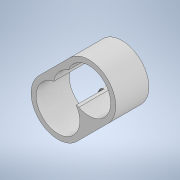
# Autodesk Inventor part: Part4
Saved by Autodesk Inventor 2020 (Build 240168000, 168)
## iProperties
Created: 2020-02-11
Part Number: Part4
Material: Generic
Document SubType Name: Modeling
Designer: atmat
Density: 1 g/cm^3
Appearance: Default
Author: atmat
Autodesk Inventor part; units mm, degrees
ref_plane "YZ Plane" through (0, 0, 0) normal (1, 0, 0) x (0, 1, 0)
ref_plane "XZ Plane" through (0, 0, 0) normal (0, 1, 0) x (-1, 0, 0)
ref_plane "XY Plane" through (0, 0, 0) normal (0, 0, 1) x (1, 0, 0)
sketch "Sketch1" plane through (0, 0, 0) normal (0, 0, 1) x (1, 0, 0)
  circle A0 centre (0, 0) radius 12.35
  circle A1 centre (7.4246, 7.4246) radius 12.2
  line L0 (-13.413, -13.413) -> (25.4094, 25.4094) construction
  line L1 (-10.6165, 0) -> (15.2552, 0) construction
  line L2 (7.4246, 7.4246) -> (15.8638, 6.41) construction
  line L3 (16.6649, 18.5138) -> (22.6753, 24.5242) construction
  circle A2 centre (15.8638, 6.41) radius 1.5
  line L4 (7.4246, 7.4246) -> (-1.0146, 8.4392) construction
  circle A3 centre (-1.0146, 8.4392) radius 1.5
  line L5 (0, 0) -> (-1.0146, 8.4392) construction
  line L6 (0, 0) -> (1.0146, -8.4392) construction
  circle A4 centre (1.0146, -8.4392) radius 1.5
  circle A5 centre (-9.8288, -9.8288) radius 12.2
  line L7 (-5.2409, -11.1828) -> (0, 0)
  point P0 (11.6813, -4.0087)
  point P1 (-0.7603, -1.6223)
  dimension "d0" = 24.7
  dimension "d1" = 24.4
  dimension "d2" = 0
  dimension "d3" = 45
  dimension "d4" = 0
  dimension "d5" = 10.5
  dimension "d20" = 8.5
  dimension "d21" = 3
  dimension "d22" = 3
  dimension "d23" = 3
  dimension "d24" = 24.4
  dimension "d25" = 24.4
  dimension "d26" = 4.5
  constraints: 18 end point, 5 centre point, 4 coincident, 4 equal length, 2 collinear, 1 horizontal, 3 other
  measures "d1" diameter of A1
  measures "d2" distance from line of point (0, 0) L0
  measures "d3" angle of L1 L0
  measures "d4" distance from line of L0 L2.start
  measures "d5" distance of point (0, 0) L2.start
  measures "d20" distance of L3.start L3.end
  measures "d21" diameter of A2
  measures "d22" diameter of A3
  measures "d23" diameter of A4
  measures "d24" diameter of A5
  measures "d25" distance of L2.start A5.centre
  measures "d26" distance from line of L7 L6.end
extrude "Extrusion1" add sketch "Sketch1" along normal blind 3 contours A0 A5 A4 L7 A1 | A0 L7 A5 A4
sketch "Sketch3" plane through (0, 0, 3) normal (0, 0, 1) x (1, 0, 0)
  circle A0 centre (0, 0) radius 12.35
  circle A1 centre (7.4246, 7.4246) radius 12.2
  line L0 (-13.413, -13.413) -> (25.4094, 25.4094) construction
  line L1 (-10.6165, 0) -> (15.2552, 0) construction
  line L2 (7.4246, 7.4246) -> (15.8638, 6.41) construction
  line L3 (16.6649, 18.5138) -> (22.6753, 24.5242) construction
  circle A2 centre (15.8638, 6.41) radius 1.5
  line L4 (7.4246, 7.4246) -> (-1.0146, 8.4392) construction
  circle A3 centre (-1.0146, 8.4392) radius 1.5
  line L5 (0, 0) -> (-1.0146, 8.4392) construction
  line L6 (0, 0) -> (1.0146, -8.4392) construction
  circle A4 centre (1.0146, -8.4392) radius 1.5
  circle A5 centre (-9.8288, -9.8288) radius 12.2
  line L7 (-5.2409, -11.1828) -> (0, 0)
  point P0 (11.6813, -4.0087)
  point P1 (-0.7603, -1.6223)
  point P2 (-0.7743, -1.6522)
  point P3 (2.1356, -7.4425)
  point P4 (2.3507, -9.1211)
  point P5 (2.146, -12.1621)
  dimension "d32" = 24.7
  dimension "d33" = 24.4
  dimension "d34" = 0
  dimension "d35" = 45
  dimension "d36" = 0
  dimension "d37" = 10.5
  dimension "d38" = 8.5
  dimension "d39" = 3
  dimension "d40" = 3
  dimension "d41" = 3
  dimension "d42" = 24.4
  dimension "d43" = 24.4
  dimension "d44" = 4.5
  constraints: 18 end point, 5 centre point, 4 coincident, 4 equal length, 2 collinear, 1 horizontal, 3 other
  measures "d33" diameter of A1
  measures "d34" distance from line of point (0, 0) L0
  measures "d35" angle of L1 L0
  measures "d36" distance from line of L0 L2.start
  measures "d37" distance of point (0, 0) L2.start
  measures "d38" distance of L3.start L3.end
  measures "d39" diameter of A2
  measures "d40" diameter of A3
  measures "d41" diameter of A4
  measures "d42" diameter of A5
  measures "d43" distance of L2.start A5.centre
  measures "d44" distance from line of L7 L6.end
extrude "Extrusion3" add sketch "Sketch3" along normal blind 15.5 contours A0 A5 A4 L7 A1 | A4 A5 picked at (2.3363, -8.2121)
sketch "Sketch4" plane through (0, 0, 3) normal (0, 0, 1) x (1, 0, 0)
  line L0 (-2.1493, -8.7099) -> (-0.8017, -5.8346)
  line L1 (-0.8017, -5.8346) -> (2.3621, -5.5639)
  line L2 (2.3621, -5.5639) -> (4.1785, -8.1686)
  line L3 (4.1785, -8.1686) -> (2.8309, -11.0439)
  line L4 (2.8309, -11.0439) -> (-0.3329, -11.3146)
  line L5 (-0.3329, -11.3146) -> (-2.1493, -8.7099)
  point P0 (0, 0)
  point P1 (1.0146, -8.4392)
  dimension "d49" = 5.5
  constraints: 12 end point, 13 other
  measures "d49" distance between parallel lines of L3 L0
extrude "Extrusion4" cut sketch "Sketch4" along normal blind 2 and the other way blind 1
sketch "Sketch5" plane through (0, 0, 18.5) normal (0, 0, 1) x (1, 0, 0)
  circle A0 centre (0, 0) radius 12.35
  circle A1 centre (7.4246, 7.4246) radius 12.2
  line L0 (-13.413, -13.413) -> (25.4094, 25.4094) construction
  line L1 (-10.6165, 0) -> (15.2552, 0) construction
  line L2 (7.4246, 7.4246) -> (15.8638, 6.41) construction
  line L3 (16.6649, 18.5138) -> (22.6753, 24.5242) construction
  circle A2 centre (15.8638, 6.41) radius 1.5
  line L4 (7.4246, 7.4246) -> (-1.0146, 8.4392) construction
  circle A3 centre (-1.0146, 8.4392) radius 1.5
  line L5 (0, 0) -> (-1.0146, 8.4392) construction
  line L6 (0, 0) -> (1.0146, -8.4392) construction
  circle A4 centre (1.0146, -8.4392) radius 1.5
  circle A5 centre (-9.8288, -9.8288) radius 12.2
  line L7 (-5.2409, -11.1828) -> (0, 0)
  line L8 (-31.042, -9.8288) -> (7.4246, 28.6378)
  line L9 (7.4246, 28.6378) -> (28.6378, 7.4246)
  line L10 (28.6378, 7.4246) -> (-9.8288, -31.042)
  line L11 (-9.8288, -31.042) -> (-31.042, -9.8288)
  circle A6 centre (-9.8288, -9.8288) radius 15
  circle A7 centre (7.4246, 7.4246) radius 15
  point P0 (11.6813, -4.0087)
  point P1 (-0.7603, -1.6223)
  point P2 (2.146, -12.1621)
  point P3 (-12.1621, 2.146)
  point P4 (-4.0087, 11.6813)
  point P5 (0.7778, -20.4354)
  point P6 (18.0312, -3.182)
  point P7 (-3.182, 18.0312)
  point P8 (-20.4354, 0.7778)
  dimension "d54" = 24.7
  dimension "d55" = 24.4
  dimension "d56" = 0
  dimension "d57" = 45
  dimension "d58" = 0
  dimension "d59" = 10.5
  dimension "d60" = 8.5
  dimension "d61" = 3
  dimension "d62" = 3
  dimension "d63" = 3
  dimension "d64" = 24.4
  dimension "d65" = 24.4
  dimension "d66" = 4.5
  dimension "d67" = 15
  dimension "d68" = 15
  dimension "d69" = 30
  dimension "d70" = 15
  constraints: 26 end point, 7 centre point, 6 coincident, 4 equal length, 2 collinear, 2 parallel, 2 perpendicular, 2 tangent, 1 horizontal, 1 point on line, 3 other
  measures "d55" diameter of A1
  measures "d56" distance from line of point (0, 0) L0
  measures "d57" angle of L1 L0
  measures "d58" distance from line of L0 L2.start
  measures "d59" distance of point (0, 0) L2.start
  measures "d60" distance of L3.start L3.end
  measures "d61" diameter of A2
  measures "d62" diameter of A3
  measures "d63" diameter of A4
  measures "d64" diameter of A5
  measures "d65" distance of L2.start A5.centre
  measures "d66" distance from line of L7 L6.end
  measures "d67" distance from line of L9 L2.start
  measures "d68" distance from line of L8 L2.start
  measures "d69" distance between parallel lines of L10 L8
  measures "d70" distance from line of A5.centre L11
extrude "Extrusion5" add sketch "Sketch5" against normal blind 18.5 contours A0 A7 A1 | A0 A6 L8 A7 | A7 L10 A6 A0 | A0 A5 A6
fillet "Fillet1" radius 3 1 edges at (-5.2409, -11.1828, 1.5)
fillet "Fillet2" radius 3 1 edges at (-0.7603, -1.6223, 9.25)
body "Solid1"
